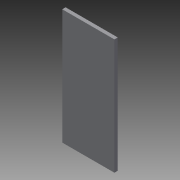
# Autodesk Inventor part: batterilock
Saved by Autodesk Inventor 2015 (Build 190159000, 159)
## iProperties
Created: 2015-12-13
Part Number: batterilock
Material: Generic
Document SubType Name: Modeling
Designer: abberik
Density: 1 g/cm^3
Appearance: Default
Author: abberik
Autodesk Inventor part; units mm, degrees
ref_plane "YZ Plane" through (0, 0, 0) normal (1, 0, 0) x (0, 1, 0)
ref_plane "XZ Plane" through (0, 0, 0) normal (0, 1, 0) x (-1, 0, 0)
ref_plane "XY Plane" through (0, 0, 0) normal (0, 0, 1) x (1, 0, 0)
sketch "Sketch1" plane through (0, 0, 0) normal (0, 1, 0) x (-1, 0, 0)
  line L0 (17.6674, 37.6255) -> (-9.3326, 37.6255)
  line L1 (-9.3326, 37.6255) -> (-9.3326, -22.1245)
  line L2 (-9.3326, -22.1245) -> (17.6674, -22.1245)
  line L3 (17.6674, -22.1245) -> (17.6674, 37.6255)
  point P0 (0, 0)
  dimension "d0" = 59.75
  dimension "d1" = 27
  constraints: 8 end point, 2 parallel, 1 horizontal, 1 perpendicular
  measures "d0" distance of L2.end L0.start
  measures "d1" distance of L1.end L2.end
extrude "Extrusion1" add sketch "Sketch1" along normal blind 1.75
body "Solid1"
